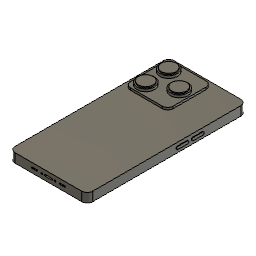
Smart_Phone_Model (Autodesk Fusion 360 design; units mm, degrees)
part number: 2026-02-12-12-44-54-767
Autodesk Fusion 360 part; units mm, degrees
sketch "Sketch1" plane through (0, 0, 0) normal (0, 1, 0) x (1, 0, 0)
  line L0 (36, 73.75) -> (-36, 73.75)
  line L1 (-36, 73.75) -> (-36, -73.75)
  line L2 (-36, -73.75) -> (36, -73.75)
  line L3 (36, -73.75) -> (36, 73.75)
  line L4 (36, 73.75) -> (-36, -73.75) construction
  line L5 (-36, 73.75) -> (36, -73.75) construction
  dimension "d1" = 72
  dimension "d2" = 147.5
  constraint horizontal L0
  constraint perpendicular L0 L1
  constraint parallel L0 L2
  constraint parallel L1 L3
  constraint coincident L4 origin
  constraint coincident L5 origin
  measures "d1" distance of L1.end L2.end
  measures "d2" distance of L0.end L1.end
extrude "Extrude1" add sketch "Sketch1" along normal blind 8.5
sketch "Sketch2" plane through (0, 8.5, 0) normal (0, 1, 0) x (-1, 0, 0)
  line L0 (-36, 73.75) -> (-36, -73.75)
  line L1 (-36, -73.75) -> (36, -73.75)
  line L2 (36, -73.75) -> (36, 73.75)
  line L3 (36, 73.75) -> (-36, 73.75)
  line L4 (36, -73.75) -> (32.5, -73.75) construction
  line L5 (32.5, -73.75) -> (32.5, -70.25) construction
  line L6 (32.5, -70.25) -> (-7, -70.25)
  line L7 (-7, -70.25) -> (-7, -29.75)
  line L8 (-7, -29.75) -> (32.5, -29.75)
  line L9 (32.5, -29.75) -> (32.5, -70.25)
  dimension "d5" = 3.5
  dimension "d6" = 3.5
  dimension "d7" = 39.5
  dimension "d8" = 40.5
  constraint coincident L1.end L2.start
  constraint perpendicular L2 L4
  constraint perpendicular L1 L5
  constraint horizontal L6
  constraint vertical L7
  constraint horizontal L8
  constraint vertical L9
  measures "d5" distance of L1.end L4.end
  measures "d6" distance of L4.end L5.end
  measures "d7" distance of L5.end L6.end
  measures "d8" distance of L5.end L8.end
extrude "Extrude2" add sketch "Sketch2" along normal blind 2 contours L6 L7 L8 L9
sketch "Sketch3" plane through (0, 10.5, 0) normal (0, 1, 0) x (-1, 0, 0)
  line L0 (32.5, -29.75) -> (-7, -29.75)
  line L1 (-7, -29.75) -> (-7, -70.25)
  line L2 (-7, -70.25) -> (32.5, -70.25)
  line L3 (32.5, -70.25) -> (32.5, -29.75)
  line L4 (32.5, -50) -> (-7, -50) construction
  line L5 (32.5, -70.25) -> (22.9, -70.25) construction
  line L6 (22.9, -70.25) -> (22.9, -60.65) construction
  circle A0 centre (22.9, -60.65) radius 8.1
  line L7 (32.5, -50) -> (2.6, -50) construction
  circle A1 centre (2.6, -50) radius 8.1
  circle A2 centre (22.9, -39.35) radius 8.1
  circle A3 centre (22.9, -60.65) radius 6.85
  circle A4 centre (22.9, -39.35) radius 6.85
  circle A5 centre (2.6, -50) radius 6.85
  dimension "d11" = 9.6
  dimension "d12" = 9.6
  dimension "d13" = 16.2
  dimension "d14" = 29.9
  dimension "d15" = 16.2
  dimension "d20" = 13.7
  dimension "d21" = 13.7
  dimension "d22" = 13.7
  constraint midpoint L3 L4.start
  constraint midpoint L1 L4.end
  constraint coincident L2.end L3.start
  constraint perpendicular L3 L5
  constraint perpendicular L5 L6
  constraint coincident L6.end A0.centre
  constraint perpendicular L3 L7
  constraint coincident L7.end A1.centre
  constraint symmetric L4 A0 A2
  constraint concentric A0 A3
  constraint concentric A2 A4
  constraint concentric A1 A5
  measures "d11" distance of L2.end L5.end
  measures "d12" distance of L5.end L6.end
  measures "d13" diameter of A0
  measures "d14" distance of L4.start L7.end
  measures "d15" diameter of A1
  measures "d20" diameter of A3
  measures "d21" diameter of A4
  measures "d22" diameter of A5
extrude "Extrude4" add sketch "Sketch3" along normal blind 2.2 contours A0 | A1 | A2 | A3 | A4 | A5
sketch "Sketch4" plane through (0, 10.5, 0) normal (0, 1, 0) x (-1, 0, 0)
extrude "Extrude5" add sketch "Sketch3" along normal blind 3.2 contours A3 | A4 | A5
fillet "Fillet1" radius 5 4 edges at (7, 9.5, -29.75) (-32.5, 9.5, -29.75) (7, 9.5, -70.25) (-32.5, 9.5, -70.25)
sketch "Sketch5" plane through (-36, 0, 0) normal (-1, 0, 0) x (0, 0, 1)
  line L0 (-73.75, 0) -> (73.75, 0)
  line L1 (73.75, 0) -> (73.75, 8.5)
  line L2 (73.75, 8.5) -> (-73.75, 8.5)
  line L3 (-73.75, 8.5) -> (-73.75, 0)
  line L4 (-73.75, 8.5) -> (-73.75, 4.25) construction
  line L5 (-73.75, 4.25) -> (-21.25, 4.25) construction
  line L6 (-12.45, 5.55) -> (-30.05, 5.55)
  line L7 (-30.05, 5.55) -> (-30.05, 2.95)
  line L8 (-30.05, 2.95) -> (-12.45, 2.95)
  line L9 (-12.45, 2.95) -> (-12.45, 5.55)
  line L10 (-12.45, 5.55) -> (-30.05, 2.95) construction
  line L11 (-30.05, 5.55) -> (-12.45, 2.95) construction
  point P0 (-21.25, 4.25)
  dimension "d27" = 52.5
  dimension "d28" = 17.6
  dimension "d29" = 2.6
  constraint coincident L2.end L3.start
  constraint midpoint L3 L4.end
  constraint perpendicular L3 L5
  constraint horizontal L6
  constraint perpendicular L6 L7
  constraint parallel L6 L8
  constraint parallel L7 L9
  constraint coincident L10 P0
  constraint coincident L11 P0
  constraint coincident P0 L5.end
  measures "d27" distance of L4.end P0
  measures "d28" distance of L7.end L8.end
  measures "d29" distance of L6.end L7.end
extrude "Extrude6" add sketch "Sketch5" along normal blind 0.5 contours L6 L7 L8 L9
fillet "Fillet2" radius 1 4 edges at (-36.25, 5.55, -12.45) (-36.25, 2.95, -12.45) (-36.25, 2.95, -30.05) (-36.25, 5.55, -30.05)
sketch "Sketch6" plane through (36, 0, 0) normal (1, 0, 0) x (0, 0, -1)
  line L0 (-73.75, 0) -> (73.75, 0)
  line L1 (73.75, 0) -> (73.75, 8.5)
  line L2 (73.75, 8.5) -> (-73.75, 8.5)
  line L3 (-73.75, 8.5) -> (-73.75, 0)
  line L4 (73.75, 4.25) -> (21.25, 4.25) construction
  line L5 (21.25, 4.25) -> (21.25, 8.5) construction
  line L6 (21.25, 4.25) -> (21.25, 0) construction
  line L7 (21.25, 4.25) -> (28.35, 4.25) construction
  line L8 (33.95, 5.55) -> (22.75, 5.55)
  line L9 (22.75, 5.55) -> (22.75, 2.95)
  line L10 (22.75, 2.95) -> (33.95, 2.95)
  line L11 (33.95, 2.95) -> (33.95, 5.55)
  line L12 (33.95, 5.55) -> (22.75, 2.95) construction
  line L13 (22.75, 5.55) -> (33.95, 2.95) construction
  line L14 (21.25, 4.25) -> (14.15, 4.25) construction
  line L15 (8.55, 5.55) -> (19.75, 5.55)
  line L16 (19.75, 5.55) -> (19.75, 2.95)
  line L17 (19.75, 2.95) -> (8.55, 2.95)
  line L18 (8.55, 2.95) -> (8.55, 5.55)
  line L19 (8.55, 5.55) -> (19.75, 2.95) construction
  line L20 (19.75, 5.55) -> (8.55, 2.95) construction
  point P0 (28.35, 4.25)
  point P1 (14.15, 4.25)
  dimension "d34" = 52.5
  dimension "d35" = 7.1
  dimension "d36" = 11.2
  dimension "d37" = 2.6
  dimension "d42" = 7.1
  dimension "d43" = 11.2
  dimension "d44" = 2.6
  constraint midpoint L1 L4.start
  constraint perpendicular L1 L4
  constraint coincident L2 L5.end
  constraint perpendicular L2 L5
  constraint coincident L0 L6.end
  constraint perpendicular L0 L6
  constraint perpendicular L6 L7
  constraint horizontal L8
  constraint perpendicular L8 L9
  constraint parallel L8 L10
  constraint parallel L9 L11
  constraint coincident L12 P0
  constraint coincident L13 P0
  constraint coincident P0 L7.end
  constraint perpendicular L6 L14
  constraint horizontal L15
  constraint perpendicular L15 L16
  constraint parallel L15 L17
  constraint parallel L16 L18
  constraint coincident L19 P1
  constraint coincident L20 P1
  constraint coincident P1 L14.end
  measures "d34" distance of L4.start L4.end
  measures "d35" distance of L4.end P0
  measures "d36" distance of L9.end L10.end
  measures "d37" distance of L8.end L9.end
  measures "d42" distance of L4.end P1
  measures "d43" distance of L16.end L17.end
  measures "d44" distance of L15.end L16.end
extrude "Extrude7" add sketch "Sketch6" along normal blind 0.5 contours L8 L9 L10 L11
fillet "Fillet3" radius 1 4 edges at (36.25, 5.55, -22.75) (36.25, 5.55, -33.95) (36.25, 2.95, -33.95) (36.25, 2.95, -22.75)
extrude "Extrude8" add sketch "Sketch6" along normal blind 0.5 contours L15 L16 L17 L18
fillet "Fillet4" radius 1 4 edges at (36.25, 5.55, -8.55) (36.25, 2.95, -8.55) (36.25, 5.55, -19.75) (36.25, 2.95, -19.75)
sketch "Sketch7" plane through (0, 0, 73.75) normal (0, 0, 1) x (1, 0, 0)
  line L0 (-36, 0) -> (36, 0)
  line L1 (36, 0) -> (36, 8.5)
  line L2 (36, 8.5) -> (-36, 8.5)
  line L3 (-36, 8.5) -> (-36, 0)
  line L4 (0, 8.5) -> (0, 0) construction
  line L5 (-3.75, 5) -> (3.75, 5)
  line L6 (3.75, 5) -> (3.75, 3.5)
  line L7 (3.75, 3.5) -> (-3.75, 3.5)
  line L8 (-3.75, 3.5) -> (-3.75, 5)
  line L9 (-3.75, 5) -> (3.75, 3.5) construction
  line L10 (3.75, 5) -> (-3.75, 3.5) construction
  line L11 (3.75, 4.25) -> (6, 4.25) construction
  circle A0 centre (6, 4.25) radius 0.75
  line L12 (6, 4.25) -> (11, 4.25) construction
  circle A1 centre (11, 4.25) radius 0.75
  line L13 (11, 4.25) -> (13, 4.25) construction
  line L14 (13, 4.25) -> (15, 4.25) construction
  circle A2 centre (13, 4.25) radius 0.75
  circle A3 centre (15, 4.25) radius 0.75
  circle A4 centre (-6, 4.25) radius 0.75
  circle A5 centre (-11, 4.25) radius 0.75
  circle A6 centre (-13, 4.25) radius 0.75
  circle A7 centre (-15, 4.25) radius 0.75
  point P0 (0, 4.25)
  dimension "d49" = 7.5
  dimension "d50" = 1.5
  dimension "d51" = 2.25
  dimension "d52" = 1.5
  dimension "d53" = 5
  dimension "d54" = 1.5
  dimension "d55" = 2
  dimension "d56" = 2
  dimension "d57" = 1.5
  dimension "d58" = 1.5
  constraint midpoint L2 L4.start
  constraint coincident L4.end origin
  constraint horizontal L5
  constraint perpendicular L5 L6
  constraint parallel L5 L7
  constraint parallel L6 L8
  constraint coincident L9 P0
  constraint coincident L10 P0
  constraint midpoint L4 P0
  constraint midpoint L6 L11.start
  constraint perpendicular L6 L11
  constraint coincident L11.end A0.centre
  constraint parallel L11 L12
  constraint coincident L12.end A1.centre
  constraint parallel L12 L13
  constraint parallel L13 L14
  constraint coincident L13.end L14.start
  constraint coincident L14.end A3.centre
  constraint symmetric L4 A0 A4
  constraint symmetric L4 A1 A5
  constraint symmetric L4 A2 A6
  constraint symmetric L4 A3 A7
  measures "d49" distance of L6.end L7.end
  measures "d50" distance of L5.end L6.end
  measures "d51" distance of L11.start L11.end
  measures "d52" diameter of A0
  measures "d53" distance of L11.end L12.end
  measures "d54" diameter of A1
  measures "d55" distance of L12.end L13.end
  measures "d56" distance of L13.end L14.end
  measures "d57" diameter of A2
  measures "d58" diameter of A3
extrude "Extrude9" cut sketch "Sketch7" against normal blind 10 contours L5 L6 L7 L8
extrude "Extrude10" cut sketch "Sketch7" against normal blind 0.5 contours A0 | A1 | A2 | A3 | A4 | A5 | A6 | A7
fillet "Fillet5" radius 1 4 edges at (-3.75, 5, 68.75) (3.75, 5, 68.75) (3.75, 3.5, 68.75) (-3.75, 3.5, 68.75)
fillet "Fillet6" radius 5 4 edges at (-36, 4.25, 73.75) (36, 4.25, 73.75) (36, 4.25, -73.75) (-36, 4.25, -73.75)
extrude "Extrude3" add sketch "Sketch3" along normal blind 2.2 contours A0 | A1 | A2 | A3 | A4 | A5
